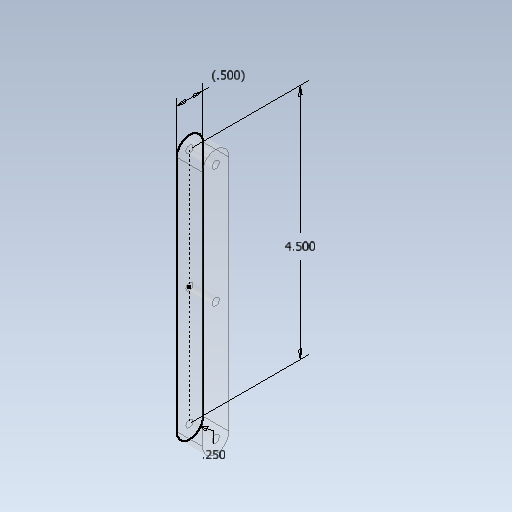
# Autodesk Inventor part: Side lexan spacer for Glock
Saved by Autodesk Inventor 2021 (Build 250183000, 183)
## iProperties
Created: 2021-02-04
Part Number: Side lexan spacer for Glock
Material: Polycarbonate, Clear
Document SubType Name: Modeling
Designer: aidan
Density: 1.2 g/cm^3
Appearance: Polycarbonate - Clear
Author: aidan
Autodesk Inventor part; units mm, degrees
ref_plane "YZ Plane" through (0, 0, 0) normal (1, 0, 0) x (0, 1, 0)
ref_plane "XZ Plane" through (0, 0, 0) normal (0, 1, 0) x (-1, 0, 0)
ref_plane "XY Plane" through (0, 0, 0) normal (0, 0, 1) x (1, 0, 0)
sketch "Sketch1" plane through (0, 0, 0) normal (1, 0, 0) x (0, 1, 0)
  line L0 (0, 0) -> (114.3, 0) construction
  line L1 (0, -6.35) -> (114.3, -6.35)
  line L2 (114.3, 6.35) -> (0, 6.35)
  arc A0 (0, 6.35) -> (0, -6.35) centre (0, 0) ccw
  arc A1 (114.3, -6.35) -> (114.3, 6.35) centre (114.3, 0) ccw
  point P0 (57.15, 0)
  dimension "d0" = 114.3
  dimension "d1" = 6.35
  dimension "d12" = 12.7
  constraints: 8 end point, 4 point on circle, 4 tangent, 2 centre point, 1 horizontal, 1 midpoint, 1 parallel
  measures "d0" distance of L0.start L0.end
  measures "d1" radius of A0
  measures "d12" distance between parallel lines of L2 L1
extrude "Extrusion1" add sketch "Sketch1" along normal blind 12.7
sketch "Sketch2" plane through (12.7, 0, 0) normal (1, 0, 0) x (0, 0, -1)
  arc A0 (6.35, 114.3) -> (-6.35, 114.3) centre (0, 114.3) ccw projected
  line L0 (-6.35, 114.3) -> (-6.35, 0) projected
  arc A1 (-6.35, 0) -> (6.35, 0) centre (0, 0) ccw projected
  line L1 (6.35, 0) -> (6.35, 114.3) projected
  circle A2 centre (0, 114.3) radius 1.7272
  circle A3 centre (0, 0) radius 1.7272
  circle A4 centre (0, 57.15) radius 1.7272
  dimension "d4" = 3.4544
  dimension "d10" = 57.15
  dimension "d11" = 6.35
  constraints: 3 centre point, 2 coincident, 2 equal radius
  measures "d4" diameter of A2
  measures "d10" distance of A4.centre A0.centre
  measures "d11" distance from line of L1 A4.centre
extrude "Extrusion2" cut sketch "Sketch2" against normal blind 12.7 contours A2 | A3 | A4
body "Solid1"
